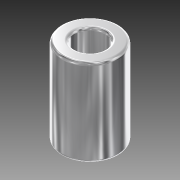
# Autodesk Inventor part: cojinete lm10uu
Saved by Autodesk Inventor 2012 SP2 (Build 160219200, 219)
## iProperties
Created: 2014-06-29
Part Number: cojinete lm10uu
Material: Default
Document SubType Name: Modeling
Designer: Principal
Density: 1 g/cm^3
Author: Principal
Autodesk Inventor part; units mm, degrees
ref_plane "YZ Plane" through (0, 0, 0) normal (1, 0, 0) x (0, 1, 0)
ref_plane "XZ Plane" through (0, 0, 0) normal (0, 1, 0) x (-1, 0, 0)
ref_plane "XY Plane" through (0, 0, 0) normal (0, 0, 1) x (1, 0, 0)
sketch "Boceto1" plane through (0, 0, 0) normal (0, 0, 1) x (1, 0, 0)
  circle A0 centre (0, 0) radius 9.5
  circle A1 centre (0, 0) radius 5
  dimension "d3" = 19
  constraints: 2 centre point, 2 coincident
  measures "d3" diameter of A0
extrude "Extrusión1" add sketch "Boceto1" along normal blind 29
fillet "Empalme1" radius 1 4 edges at (-9.5, 0, 29) (-5, 0, 29) (-9.5, 0, 0) (-5, 0, 0)
